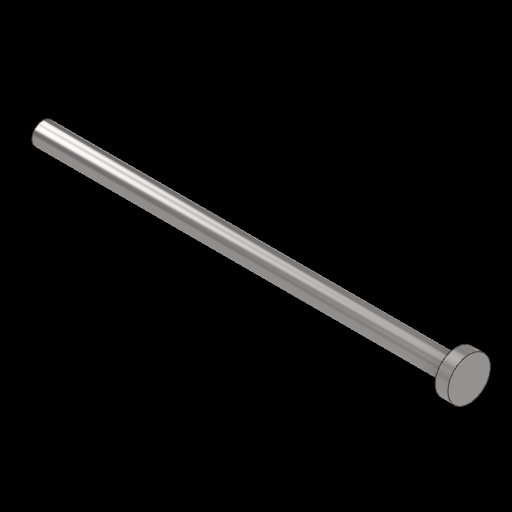
# Autodesk Inventor part: Marks - R80/5,2/100
Saved by Autodesk Inventor 2024 (Build 280153000, 153)
## iProperties
Created: 2023-06-30
Part Number: Marks - R80/5,2/100
Material: Edelstahl, austenitisch
Document SubType Name: Modeling
Designer: buchmannmartin
Density: 8 g/cm^3
Appearance: Halbpoliert
Catalog Web Link: https://www.marks-gmbh.de/shop/werkstattbedarf/auswerfer-schneidstempel/auswerferstifte/form-ah
Description: Auswerfer DIN1530-AH 1.2067/1.2516 geh.
Vendor: Makrs Eisenberg
Mass: 18.3676 g
Surface Area: 18.3388 cm^2
Volume: 2.29595 cm^3
Author: buchmannmartin
Autodesk Inventor part; units mm, degrees
ref_plane "YZ Plane" through (0, 0, 0) normal (1, 0, 0) x (0, 1, 0)
ref_plane "XZ Plane" through (0, 0, 0) normal (0, 1, 0) x (-1, 0, 0)
ref_plane "XY Plane" through (0, 0, 0) normal (0, 0, 1) x (1, 0, 0)
sketch "Skizze1" plane through (0, 0, 0) normal (0, 0, 1) x (1, 0, 0)
  line L0 (0, 0) -> (0, 5)
  line L1 (0, 5) -> (-3, 5)
  line L2 (-3, 5) -> (-3, 2.9)
  line L3 (-3.3, 2.6) -> (-100, 2.6)
  line L4 (-100, 2.6) -> (-100, 0)
  line L5 (-100, 0) -> (0, 0)
  arc A0 (-3.3, 2.6) -> (-3, 2.9) centre (-3.3, 2.9) ccw
  dimension "d0" = 5.2
  dimension "d1" = 100
  dimension "d2" = 10
  dimension "d3" = 3
  dimension "d4" = 0.3
  constraints: 12 end point, 5 perpendicular, 2 point on circle, 2 tangent, 1 centre point, 1 vertical
  measures "d0" diameter of L3 L5
  measures "d1" distance of L4.end L0.start
  measures "d2" diameter of L1 L5
  measures "d3" distance of L0.end L1.end
  measures "d4" radius of A0
revolve "Umdrehung1" add sketch "Skizze1" angle 360 about axis through (-100, 0, 0) along (1, 0, 0)
